Autodesk Inventor part; units mm, degrees
(part 3 of 3)
sketch "Sketch25" plane through (0, 0, 0) normal (-1, 0, 0) x (0, 0, 1)
  circle A0 centre (0, 0) radius 104.7779
  spline S0 degree 2 poles (-63.7511, 55.753) (-62.5258, 54.8622) (-61.3256, 52.5646) (-61.2745, 51.3467) knots 0 0 0 1 2 2 2
  spline S1 degree 2 poles (-61.2745, 51.3467) (-61.2331, 49.8915) (-62.16, 47.3283) (-63.3801, 45.6501) knots 0 0 0 1 2 2 2
  line L0 (-63.3801, 45.6501) -> (-66.8079, 40.9352)
  line L1 (-66.8079, 40.9352) -> (-83.2435, 52.884)
  line L2 (-83.2435, 52.884) -> (-80.0771, 57.2393)
  spline S2 degree 2 poles (-80.0771, 57.2393) (-78.799, 58.9974) (-77.2944, 60.5909) (-76.2739, 61.0705) knots 0 0 0 1 2 2 2
  spline S3 degree 2 poles (-76.2739, 61.0705) (-75.159, 61.624) (-73.0366, 61.3229) (-71.9978, 60.5676) knots 0 0 0 1 2 2 2
  spline S4 degree 2 poles (-71.9978, 60.5676) (-70.839, 59.7252) (-69.8918, 57.1636) (-70.1567, 55.7071) knots 0 0 0 1 2 2 2
  line L3 (-70.1567, 55.7071) -> (-70.0768, 55.649)
  spline S5 degree 2 poles (-70.0768, 55.649) (-68.6121, 56.8236) (-65.3228, 56.8956) (-63.7511, 55.753) knots 0 0 0 1 2 2 2
  spline S6 degree 2 poles (-65.3137, 53.4077) (-66.246, 54.0855) (-67.832, 54.4242) (-68.8392, 53.9349) knots 0 0 0 1 2 2 2
  spline S7 degree 2 poles (-68.8392, 53.9349) (-69.4832, 53.6092) (-70.5339, 52.5) (-71.3569, 51.3679) knots 0 0 0 1 2 2 2
  line L4 (-71.3569, 51.3679) -> (-73.158, 48.8906)
  line L5 (-73.158, 48.8906) -> (-67.0845, 44.4751)
  line L6 (-67.0845, 44.4751) -> (-65.7967, 46.2466)
  spline S8 degree 2 poles (-65.7967, 46.2466) (-64.7509, 47.685) (-63.8166, 49.5302) (-63.778, 50.4794) knots 0 0 0 1 2 2 2
  spline S9 degree 2 poles (-63.778, 50.4794) (-63.7721, 51.4116) (-64.4479, 52.7783) (-65.3137, 53.4077) knots 0 0 0 1 2 2 2
  spline S10 degree 2 poles (-73.3472, 58.0674) (-73.9333, 58.4934) (-75.1028, 58.7329) (-75.6754, 58.4774) knots 0 0 0 1 2 2 2
  spline S11 degree 2 poles (-75.6754, 58.4774) (-76.3557, 58.1576) (-77.4282, 56.9625) (-78.2706, 55.8038) knots 0 0 0 1 2 2 2
  line L7 (-78.2706, 55.8038) -> (-79.7908, 53.7127)
  line L8 (-79.7908, 53.7127) -> (-74.9827, 50.2171)
  line L9 (-74.9827, 50.2171) -> (-73.1816, 52.6945)
  spline S12 degree 2 poles (-73.1816, 52.6945) (-72.436, 53.72) (-71.9423, 54.8472) (-71.8976, 55.6088) knots 0 0 0 1 2 2 2
  spline S13 degree 2 poles (-71.8976, 55.6088) (-71.8493, 56.3473) (-72.5747, 57.5057) (-73.3472, 58.0674) knots 0 0 0 1 2 2 2
  line L10 (-56.7812, 53.9458) -> (-70.4397, 68.9906)
  line L11 (-70.4397, 68.9906) -> (-61.0276, 77.5355)
  line L12 (-61.0276, 77.5355) -> (-59.4116, 75.7555)
  line L13 (-59.4116, 75.7555) -> (-66.8243, 69.0259)
  line L14 (-66.8243, 69.0259) -> (-63.0831, 64.905)
  line L15 (-63.0831, 64.905) -> (-56.1703, 71.1808)
  line L16 (-56.1703, 71.1808) -> (-54.5543, 69.4008)
  line L17 (-54.5543, 69.4008) -> (-61.4671, 63.125)
  line L18 (-61.4671, 63.125) -> (-56.3978, 57.541)
  line L19 (-56.3978, 57.541) -> (-48.9851, 64.2707)
  line L20 (-48.9851, 64.2707) -> (-47.3691, 62.4907)
  line L21 (-47.3691, 62.4907) -> (-56.7812, 53.9458)
  spline S14 degree 2 poles (-39.8769, 66.74) (-41.7719, 65.6096) (-44.903, 64.8157) (-46.4142, 64.6812) knots 0 0 0 1 2 2 2
  line L22 (-46.4142, 64.6812) -> (-48.152, 67.5945)
  line L23 (-48.152, 67.5945) -> (-47.9823, 67.6957)
  spline S15 degree 2 poles (-47.9823, 67.6957) (-46.1957, 67.3042) (-42.588, 67.8455) (-41.2445, 68.6469) knots 0 0 0 1 2 2 2
  spline S16 degree 2 poles (-41.2445, 68.6469) (-39.3212, 69.7942) (-38.3086, 72.5647) (-39.0932, 73.8799) knots 0 0 0 1 2 2 2
  spline S17 degree 2 poles (-39.0932, 73.8799) (-39.7174, 74.9265) (-41.5258, 75.6117) (-42.8371, 75.2706) knots 0 0 0 1 2 2 2
  spline S18 degree 2 poles (-42.8371, 75.2706) (-43.7781, 75.016) (-45.3072, 74.5258) (-46.4631, 74.1814) knots 0 0 0 1 2 2 2
  spline S19 degree 2 poles (-46.4631, 74.1814) (-47.5116, 73.8819) (-49.3702, 73.7512) (-50.2676, 74.002) knots 0 0 0 1 2 2 2
  spline S20 degree 2 poles (-50.2676, 74.002) (-51.1508, 74.2613) (-52.6727, 75.4626) (-53.2801, 76.4808) knots 0 0 0 1 2 2 2
  spline S21 degree 2 poles (-53.2801, 76.4808) (-54.5454, 78.6021) (-52.9486, 83.4469) (-50.3889, 84.9737) knots 0 0 0 1 2 2 2
  spline S22 degree 2 poles (-50.3889, 84.9737) (-48.9181, 85.851) (-45.9701, 86.8233) (-44.5239, 86.9382) knots 0 0 0 1 2 2 2
  line L24 (-44.5239, 86.9382) -> (-42.8706, 84.1664)
  line L25 (-42.8706, 84.1664) -> (-43.0403, 84.0652)
  spline S23 degree 2 poles (-43.0403, 84.0652) (-44.3302, 84.3311) (-47.6071, 83.9103) (-49.0355, 83.0583) knots 0 0 0 1 2 2 2
  spline S24 degree 2 poles (-49.0355, 83.0583) (-50.6477, 82.0967) (-51.7391, 79.3941) (-51.0052, 78.1637) knots 0 0 0 1 2 2 2
  spline S25 degree 2 poles (-51.0052, 78.1637) (-50.3472, 77.0607) (-48.3889, 76.4456) (-47.1087, 76.8066) knots 0 0 0 1 2 2 2
  spline S26 degree 2 poles (-47.1087, 76.8066) (-46.2552, 77.0473) (-43.8161, 77.8119) (-42.9825, 78.0216) knots 0 0 0 1 2 2 2
  spline S27 degree 2 poles (-42.9825, 78.0216) (-40.8574, 78.5413) (-37.8643, 77.3164) (-36.8942, 75.6901) knots 0 0 0 1 2 2 2
  spline S28 degree 2 poles (-36.8942, 75.6901) (-36.2784, 74.6578) (-35.9318, 72.1802) (-36.268, 71.0401) knots 0 0 0 1 2 2 2
  spline S29 degree 2 poles (-36.268, 71.0401) (-36.6468, 69.7788) (-38.2789, 67.6932) (-39.8769, 66.74) knots 0 0 0 1 2 2 2
  line L26 (-26.9235, 73.3338) -> (-32.8028, 90.2575)
  line L27 (-32.8028, 90.2575) -> (-39.2425, 88.0203)
  line L28 (-39.2425, 88.0203) -> (-40.0315, 90.2913)
  line L29 (-40.0315, 90.2913) -> (-24.6011, 95.6519)
  line L30 (-24.6011, 95.6519) -> (-23.8121, 93.3809)
  line L31 (-23.8121, 93.3809) -> (-30.2518, 91.1437)
  line L32 (-30.2518, 91.1437) -> (-24.3725, 74.22)
  line L33 (-24.3725, 74.22) -> (-26.9235, 73.3338)
  spline S30 degree 2 poles (-1.5556, 77.7301) (-3.7618, 77.6876) (-6.8747, 78.5499) (-8.2539, 79.1822) knots 0 0 0 1 2 2 2
  line L34 (-8.2539, 79.1822) -> (-8.3192, 82.5737)
  line L35 (-8.3192, 82.5737) -> (-8.1217, 82.5775)
  spline S31 degree 2 poles (-8.1217, 82.5775) (-6.764, 81.3519) (-3.3623, 80.034) (-1.7982, 80.0642) knots 0 0 0 1 2 2 2
  spline S32 degree 2 poles (-1.7982, 80.0642) (0.4408, 80.1073) (2.6934, 82.0118) (2.6639, 83.543) knots 0 0 0 1 2 2 2
  spline S33 degree 2 poles (2.6639, 83.543) (2.6404, 84.7613) (1.4094, 86.2528) (0.1015, 86.6064) knots 0 0 0 1 2 2 2
  spline S34 degree 2 poles (0.1015, 86.6064) (-0.842, 86.8517) (-2.4131, 87.1838) (-3.5877, 87.4576) knots 0 0 0 1 2 2 2
  spline S35 degree 2 poles (-3.5877, 87.4576) (-4.6468, 87.7172) (-6.3258, 88.5248) (-6.9809, 89.1874) knots 0 0 0 1 2 2 2
  spline S36 degree 2 poles (-6.9809, 89.1874) (-7.6195, 89.8504) (-8.3459, 91.648) (-8.3687, 92.8334) knots 0 0 0 1 2 2 2
  spline S37 degree 2 poles (-8.3687, 92.8334) (-8.4163, 95.303) (-4.6282, 98.7194) (-1.6483, 98.7768) knots 0 0 0 1 2 2 2
  spline S38 degree 2 poles (-1.6483, 98.7768) (0.0639, 98.8098) (3.1063, 98.1932) (4.4193, 97.5761) knots 0 0 0 1 2 2 2
  line L36 (4.4193, 97.5761) -> (4.4815, 94.3492)
  line L37 (4.4815, 94.3492) -> (4.2839, 94.3454)
  spline S39 degree 2 poles (4.2839, 94.3454) (3.2954, 95.2158) (0.2407, 96.4745) (-1.4221, 96.4424) knots 0 0 0 1 2 2 2
  spline S40 degree 2 poles (-1.4221, 96.4424) (-3.299, 96.4063) (-5.5864, 94.5999) (-5.5588, 93.1676) knots 0 0 0 1 2 2 2
  spline S41 degree 2 poles (-5.5588, 93.1676) (-5.5341, 91.8834) (-4.1381, 90.3786) (-2.8473, 90.0576) knots 0 0 0 1 2 2 2
  spline S42 degree 2 poles (-2.8473, 90.0576) (-1.9867, 89.8436) (0.5107, 89.2988) (1.3387, 89.0677) knots 0 0 0 1 2 2 2
  spline S43 degree 2 poles (1.3387, 89.0677) (3.442, 88.466) (5.4345, 85.9186) (5.471, 84.0253) knots 0 0 0 1 2 2 2
  spline S44 degree 2 poles (5.471, 84.0253) (5.4941, 82.8234) (4.5672, 80.4998) (3.7102, 79.6762) knots 0 0 0 1 2 2 2
  spline S45 degree 2 poles (3.7102, 79.6762) (2.7559, 78.7685) (0.3048, 77.766) (-1.5556, 77.7301) knots 0 0 0 1 2 2 2
  line L38 (22.7653, 75.0801) -> (20.1187, 75.6172)
  line L39 (20.1187, 75.6172) -> (22.0969, 85.3644)
  line L40 (22.0969, 85.3644) -> (12.9307, 87.2247)
  line L41 (12.9307, 87.2247) -> (10.9524, 77.4775)
  line L42 (10.9524, 77.4775) -> (8.3058, 78.0147)
  line L43 (8.3058, 78.0147) -> (12.3475, 97.9287)
  line L44 (12.3475, 97.9287) -> (14.9941, 97.3915)
  line L45 (14.9941, 97.3915) -> (13.4088, 89.5808)
  line L46 (13.4088, 89.5808) -> (22.5751, 87.7205)
  line L47 (22.5751, 87.7205) -> (24.1603, 95.5312)
  line L48 (24.1603, 95.5312) -> (26.8069, 94.9941)
  line L49 (26.8069, 94.9941) -> (22.7653, 75.0801)
  line L50 (33.1213, 70.8467) -> (25.8325, 73.8179)
  line L51 (25.8325, 73.8179) -> (26.6157, 75.7392)
  line L52 (26.6157, 75.7392) -> (29.0097, 74.7633)
  line L53 (29.0097, 74.7633) -> (35.1138, 89.7374)
  line L54 (35.1138, 89.7374) -> (32.7197, 90.7133)
  line L55 (32.7197, 90.7133) -> (33.503, 92.6346)
  line L56 (33.503, 92.6346) -> (40.7917, 89.6634)
  line L57 (40.7917, 89.6634) -> (40.0085, 87.7421)
  line L58 (40.0085, 87.7421) -> (37.6145, 88.718)
  line L59 (37.6145, 88.718) -> (31.5105, 73.7439)
  line L60 (31.5105, 73.7439) -> (33.9045, 72.768)
  line L61 (33.9045, 72.768) -> (33.1213, 70.8467)
  line L62 (49.4722, 61.1263) -> (46.5084, 63.002)
  line L63 (46.5084, 63.002) -> (45.4057, 73.2683)
  line L64 (45.4057, 73.2683) -> (42.7898, 74.9239)
  line L65 (42.7898, 74.9239) -> (38.466, 68.0919)
  line L66 (38.466, 68.0919) -> (36.1841, 69.5362)
  line L67 (36.1841, 69.5362) -> (47.0508, 86.7064)
  line L68 (47.0508, 86.7064) -> (51.4755, 83.906)
  spline S46 degree 2 poles (51.4755, 83.906) (52.9504, 82.9726) (54.7376, 81.3933) (55.2722, 80.2365) knots 0 0 0 1 2 2 2
  spline S47 degree 2 poles (55.2722, 80.2365) (55.8068, 79.0797) (55.6968, 76.5964) (54.8426, 75.2468) knots 0 0 0 1 2 2 2
  spline S48 degree 2 poles (54.8426, 75.2468) (53.6537, 73.3683) (50.1221, 72.0373) (48.0927, 72.4642) knots 0 0 0 1 2 2 2
  line L69 (48.0927, 72.4642) -> (49.4722, 61.1263)
  spline S49 degree 2 poles (52.3487, 76.5717) (52.8243, 77.3231) (53.0264, 78.8126) (52.7076, 79.5405) knots 0 0 0 1 2 2 2
  spline S50 degree 2 poles (52.7076, 79.5405) (52.4232, 80.1688) (51.2965, 81.2521) (50.3503, 81.8509) knots 0 0 0 1 2 2 2
  line L70 (50.3503, 81.8509) -> (48.0823, 83.2863)
  line L71 (48.0823, 83.2863) -> (43.9962, 76.8301)
  line L72 (43.9962, 76.8301) -> (45.9999, 75.562)
  spline S51 degree 2 poles (45.9999, 75.562) (46.9878, 74.9368) (48.7803, 74.2896) (49.6664, 74.4888) knots 0 0 0 1 2 2 2
  spline S52 degree 2 poles (49.6664, 74.4888) (50.4667, 74.6448) (51.7852, 75.6812) (52.3487, 76.5717) knots 0 0 0 1 2 2 2
  line L73 (53.9025, 56.5441) -> (66.4894, 69.2936)
  line L74 (66.4894, 69.2936) -> (61.638, 74.0831)
  line L75 (61.638, 74.0831) -> (63.3271, 75.7939)
  line L76 (63.3271, 75.7939) -> (74.9516, 64.3177)
  line L77 (74.9516, 64.3177) -> (73.2625, 62.6068)
  line L78 (73.2625, 62.6068) -> (68.4112, 67.3963)
  line L79 (68.4112, 67.3963) -> (55.8243, 54.6468)
  line L80 (55.8243, 54.6468) -> (53.9025, 56.5441)
  spline S53 degree 2 poles (64.6417, 43.1954) (63.4171, 45.0309) (62.4661, 48.1179) (62.2555, 49.6204) knots 0 0 0 1 2 2 2
  line L81 (62.2555, 49.6204) -> (65.0773, 51.503)
  line L82 (65.0773, 51.503) -> (65.187, 51.3386)
  spline S54 degree 2 poles (65.187, 51.3386) (64.8862, 49.5346) (65.609, 45.9588) (66.4772, 44.6575) knots 0 0 0 1 2 2 2
  spline S55 degree 2 poles (66.4772, 44.6575) (67.7201, 42.7945) (70.5382, 41.9232) (71.8122, 42.7731) knots 0 0 0 1 2 2 2
  spline S56 degree 2 poles (71.8122, 42.7731) (72.8258, 43.4493) (73.4189, 45.2901) (73.012, 46.5824) knots 0 0 0 1 2 2 2
  spline S57 degree 2 poles (73.012, 46.5824) (72.7103, 47.5094) (72.1434, 49.0118) (71.7411, 50.1489) knots 0 0 0 1 2 2 2
  spline S58 degree 2 poles (71.7411, 50.1489) (71.3891, 51.1809) (71.1647, 53.0305) (71.3699, 53.9394) knots 0 0 0 1 2 2 2
  spline S59 degree 2 poles (71.3699, 53.9394) (71.5843, 54.8346) (72.7072, 56.4152) (73.6935, 57.0732) knots 0 0 0 1 2 2 2
  spline S60 degree 2 poles (73.6935, 57.0732) (75.7482, 58.444) (80.6674, 57.0938) (82.3215, 54.6145) knots 0 0 0 1 2 2 2
  spline S61 degree 2 poles (82.3215, 54.6145) (83.2719, 53.1899) (84.3919, 50.2947) (84.5796, 48.8562) knots 0 0 0 1 2 2 2
  line L83 (84.5796, 48.8562) -> (81.8948, 47.065)
  line L84 (81.8948, 47.065) -> (81.7851, 47.2293)
  spline S62 degree 2 poles (81.7851, 47.2293) (81.9856, 48.531) (81.3999, 51.7826) (80.4769, 53.1661) knots 0 0 0 1 2 2 2
  spline S63 degree 2 poles (80.4769, 53.1661) (79.4351, 54.7277) (76.6808, 55.6812) (75.4891, 54.8862) knots 0 0 0 1 2 2 2
  spline S64 degree 2 poles (75.4891, 54.8862) (74.4207, 54.1733) (73.9052, 52.1865) (74.3304, 50.9261) knots 0 0 0 1 2 2 2
  spline S65 degree 2 poles (74.3304, 50.9261) (74.6139, 50.0859) (75.5007, 47.6885) (75.7521, 46.8665) knots 0 0 0 1 2 2 2
  spline S66 degree 2 poles (75.7521, 46.8665) (76.3785, 44.7704) (75.3063, 41.7193) (73.731, 40.6683) knots 0 0 0 1 2 2 2
  spline S67 degree 2 poles (73.731, 40.6683) (72.7311, 40.0012) (70.2741, 39.5299) (69.1186, 39.8081) knots 0 0 0 1 2 2 2
  spline S68 degree 2 poles (69.1186, 39.8081) (67.8397, 40.1228) (65.6744, 41.6475) (64.6417, 43.1954) knots 0 0 0 1 2 2 2
  constraints: 1 centre point, 1 coincident, 1 other
sketch "Sketch26" plane through (25.4, 0, 0) normal (1, 0, 0) x (0, 0, -1)
  circle A0 centre (0, 0) radius 104.7779 projected
extrude "Extrusion16" add sketch "Sketch25" against normal blind 2.54 contours S0 S1 L0 L1 L2 S2 S3 S4 L3 S5 | L10 L11 L12 L13 L14 L15 L16 L17 L18 L19 L20 L21 | S14 L22 L23 S15 S16 S17 S18 S19 S20 S21 S22 L24 L25 S23 S24 S25 S26 S27 S28 S29 | L26 L27 L28 L29 L30 L31 L32 L33 | S30 L34 L35 S31 S32 S33 S34 S35 S36 S37 S38 L36 L37 S39 S40 S41 S42 S43 S44 S45 | L38 L39 L40 L41 L42 L43 L44 L45 L46 L47 L48 L49 | L50 L51 L52 L53 L54 L55 L56 L57 L58 L59 L60 L61 | L62 L63 L64 L65 L66 L67 L68 S46 S47 S48 L69 | L73 L74 L75 L76 L77 L78 L79 L80 | S53 L81 L82 S54 S55 S56 S57 S58 S59 S60 S61 L83 L84 S62 S63 S64 S65 S66 S67 S68
sketch "Sketch27" plane through (0, 0, 0) normal (-1, 0, 0) x (0, 0, 1)
  circle A0 centre (0, 0) radius 104.7779
  constraints: 1 centre point, 1 coincident, 1 other
sketch "Sketch28" plane through (0, 0, 0) normal (-1, 0, 0) x (0, 0, 1)
  point P0 (0, 0)
body "Solid1"
